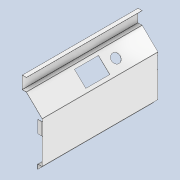
# Autodesk Inventor part: Carcaza_blanca_frontal
Saved by Autodesk Inventor 2021 (Build 250183000, 183)
## iProperties
Created: 2021-04-15
Part Number: Carcaza_blanca_frontal
Material: Genérico
Document SubType Name: Chapa
Designer: Admin
Density: 1 g/cm^3
Sheet Metal Rule: Por defecto_mm
Appearance: Blanco
Author: Admin
Autodesk Inventor part; units mm, degrees
ref_plane "YZ Plane" through (0, 0, 0) normal (1, 0, 0) x (0, 1, 0)
ref_plane "XZ Plane" through (0, 0, 0) normal (0, 1, 0) x (-1, 0, 0)
ref_plane "XY Plane" through (0, 0, 0) normal (0, 0, 1) x (1, 0, 0)
sketch "Boceto1" plane through (0, 0, 0) normal (1, 0, 0) x (0, 1, 0)
  line L0 (0, 0) -> (189.4, 0)
  line L1 (189.4, 0) -> (189.4, -527.58)
  line L2 (189.4, -527.58) -> (0, -527.58)
  line L3 (0, -527.58) -> (0, 0)
  dimension "d0" = 189.4
  dimension "d1" = 527.58
  measures "d0" distance of L1.end L2.end
  measures "d1" distance of L0.end L1.end
extrude "Placa1" add sketch "Boceto1" along normal blind 0.92
sketch "Boceto2" plane through (0.92, 0.92, -527.58) normal (0, -1, 0) x (-1, 0, 0)
  line L0 (0, 527.58) -> (0, 0)
  line L1 (0, 0) -> (21.6, 0)
  line L2 (21.6, 0) -> (21.6, 527.58)
  line L3 (21.6, 527.58) -> (0, 527.58)
  constraints: 6 end point, 1 horizontal, 1 perpendicular, 1 vertical
edge flange "Pestaña1" height 21.6 angle 90 thickness 0.92 bend radius 0.92 thickness toward (0, -1, 0) relief straight relief width 0.92 relief depth 0.46 edges at (0.92, 0, -263.79) wall of the first edge with corners at (0.92, 0.92, 0) (0.92, 0.92, -527.58) (-20.68, 0.92, -527.58) (-20.68, 0.92, 0)
bend "Doblez1"
corner "Esquina1"
sketch "Boceto3" plane through (-19.76, 0.92, 0) normal (-1, 0, 0) x (0, 1, 0)
  line L0 (0, -527.58) -> (0, 0)
  line L1 (0, 0) -> (-21.6, 0)
  line L2 (-21.6, 0) -> (-21.6, -527.58)
  line L3 (-21.6, -527.58) -> (0, -527.58)
  constraints: 8 end point
edge flange "Pestaña2" height 21.6 angle 90 thickness 0.92 bend radius 0.92 thickness toward (-1, 0, 0) relief straight relief width 0.92 relief depth 0.46 edges at (-20.68, 0.92, -263.79) wall of the first edge with corners at (-19.76, 0.92, -527.58) (-19.76, 0.92, 0) (-19.76, -20.68, 0) (-19.76, -20.68, -527.58)
bend "Doblez2"
corner "Esquina2"
sketch "Boceto4" plane through (0.2822, 188.737, 0) normal (0.6932761, 0.7206721, 0) x (0.7206721, -0.6932761, 0)
  line L0 (0, -527.58) -> (0, 0)
  line L1 (0, 0) -> (-100.563, 0)
  line L2 (-100.563, 0) -> (-100.563, -527.58)
  line L3 (-100.563, -527.58) -> (0, -527.58)
  constraints: 6 end point, 1 horizontal, 1 perpendicular, 1 vertical
edge flange "Pestaña3" height 100.563 angle 46.11 thickness 0.92 bend radius 0.92 thickness toward (0.6932761, 0.7206721, 0) relief straight relief width 0.92 relief depth 0.46 edges at (0.92, 189.4, -263.79) wall of the first edge with corners at (0.2822, 188.737, -527.58) (0.2822, 188.737, 0) (-72.1908, 258.4549, 0) (-72.1908, 258.4549, -527.58)
bend "Doblez3"
corner "Esquina3"
sketch "Boceto5" plane through (-71.553, 258.1979, 0) normal (0, 1, 0) x (1, 0, 0)
  line L0 (0, -527.58) -> (0, 0)
  line L1 (0, 0) -> (-20, 0)
  line L2 (-20, 0) -> (-20, -527.58)
  line L3 (-20, -527.58) -> (0, -527.58)
  constraints: 6 end point, 1 horizontal, 1 perpendicular, 1 vertical
edge flange "Pestaña4" height 20 angle 43.89 thickness 0.92 bend radius 0.92 thickness toward (0, 1, 0) relief straight relief width 0.92 relief depth 0.46 edges at (-71.553, 259.1179, -263.79) wall of the first edge with corners at (-71.553, 258.1979, -527.58) (-71.553, 258.1979, 0) (-91.553, 258.1979, 0) (-91.553, 258.1979, -527.58)
bend "Doblez4"
corner "Esquina4"
sketch "Boceto6" plane through (-90.633, 258.1979, 0) normal (-1, 0, 0) x (0, -1, 0)
  line L0 (0, -527.58) -> (0, 0)
  line L1 (0, 0) -> (-58.71, 0)
  line L2 (-58.71, 0) -> (-58.71, -527.58)
  line L3 (-58.71, -527.58) -> (0, -527.58)
  constraints: 6 end point, 1 horizontal, 1 perpendicular, 1 vertical
edge flange "Pestaña5" height 58.71 angle 90 thickness 0.92 bend radius 0.92 thickness toward (-1, 0, 0) relief straight relief width 0.92 relief depth 0.46 edges at (-91.553, 259.1179, -263.79) wall of the first edge with corners at (-90.633, 258.1979, -527.58) (-90.633, 258.1979, 0) (-90.633, 316.9079, 0) (-90.633, 316.9079, -527.58)
bend "Doblez5"
corner "Esquina5"
sketch "Boceto7" plane through (-91.553, 315.9879, -527.58) normal (0, 1, 0) x (1, 0, 0)
  line L0 (0, 527.58) -> (0, 0)
  line L1 (0, 0) -> (20, 0)
  line L2 (20, 0) -> (20, 527.58)
  line L3 (20, 527.58) -> (0, 527.58)
  constraints: 6 end point, 1 horizontal, 1 perpendicular, 1 vertical
edge flange "Pestaña6" height 20 angle 90 thickness 0.92 bend radius 0.92 thickness toward (0, 1, 0) relief straight relief width 0.92 relief depth 0.46 edges at (-91.553, 316.9079, -263.79) wall of the first edge with corners at (-91.553, 315.9879, 0) (-91.553, 315.9879, -527.58) (-71.553, 315.9879, -527.58) (-71.553, 315.9879, 0)
bend "Doblez6"
corner "Esquina6"
sketch "Boceto8" plane through (0, 1.84, 0) normal (0, 0, 1) x (1, 0, 0)
  line L0 (0.92, 186.7769) -> (0.92, 0)
  line L1 (0.92, 174.636) -> (-19.08, 174.636)
  line L2 (-19.08, 174.636) -> (-19.08, 118.6032)
  line L3 (-19.08, 118.6032) -> (0.92, 118.6032)
  line L4 (0.92, 118.6032) -> (0.92, 174.636)
  point P0 (0, -1.84)
  dimension "d63" = 20
  measures "d63" distance of L3.end L2.end
sheet face with bend "Cara2" sketch "Boceto8" thickness 0.92 toward (0, 0, -1) bend radius 0.92 relief straight relief width 0.92 relief depth 0.46
bend "Doblez7"
sketch "Boceto9" plane through (0, 1.84, -527.58) normal (0, 0, -1) x (-1, 0, 0)
  line L0 (-0.92, 174.636) -> (-0.92, 118.6032)
  line L1 (19.08, 174.636) -> (19.08, 118.6032)
  line L2 (-0.92, 174.636) -> (19.08, 174.636)
  line L3 (19.08, 174.636) -> (19.08, 118.6032)
  line L4 (19.08, 118.6032) -> (-0.92, 118.6032)
  line L5 (-0.92, 118.6032) -> (-0.92, 174.636)
  point P0 (0, -1.84)
sheet face with bend "Cara3" sketch "Boceto9" thickness 0.92 toward (0, 0, 1) bend radius 0.92 relief straight relief width 0.92 relief depth 0.46
bend "Doblez8"
sketch "Boceto10" plane through (0.3556, 189.9429, 0) normal (0.6932761, 0.7206721, 0) x (0.7206721, -0.6932761, 0)
  line L0 (0, 527.58) -> (0, 0) projected
  line L1 (-100.3142, 0) -> (-100.3142, 527.58) projected
  line L2 (-14, 263.79) -> (-14, 318.59)
  line L3 (-14, 318.59) -> (-85.6, 318.59)
  line L4 (-85.6, 318.59) -> (-85.6, 208.99)
  line L5 (-85.6, 208.99) -> (-14, 208.99)
  line L6 (-14, 208.99) -> (-14, 263.79)
  line L7 (-49.8, 263.79) -> (-49.8, 371.79)
  circle A0 centre (-49.8, 371.79) radius 20
  point P0 (131.4266, 0)
  dimension "d75" = 54.8
  dimension "d76" = 71.6
  dimension "d77" = 109.6
  dimension "d78" = 71.6
  dimension "d81" = 108
  dimension "d82" = 40
  constraints: 12 end point, 2 perpendicular, 1 centre point, 1 coincident, 1 point on line, 1 vertical
  measures "d75" distance of L2.start L2.end
  measures "d76" distance of L2.end L3.end
  measures "d77" distance of L3.end L4.end
  measures "d78" distance of L4.end L5.end
  measures "d81" distance of L7.start L7.end
  measures "d82" diameter of A0
extrude "Extrusión1" cut sketch "Boceto10" against normal blind 10
equation "\"d2\" = Grosor"
equation "\"d3\" = Anchura_desahogo_plegado"
equation "\"d4\" = Profundidad_desahogo_plegado"
equation "\"d5\" = Remanente_mínimo"
equation "\"d6\" = Radiodetransición"
equation "\"d9\" = Radio_pliegue"
equation "\"d10\" = Tamaño_destalonado"
equation "\"d11\" = TamañoSeparación"
equation "\"d12\" = Tamaño_de_radio_de_Jacobi"
equation "\"d13\" = Anchura_desahogo_plegado"
equation "\"d14\" = Profundidad_desahogo_plegado"
equation "\"d15\" = Remanente_mínimo"
equation "\"d16\" = Radiodetransición"
equation "\"d19\" = Radio_pliegue"
equation "\"d20\" = Tamaño_destalonado"
equation "\"d21\" = TamañoSeparación"
equation "\"d22\" = Tamaño_de_radio_de_Jacobi"
equation "\"d23\" = Anchura_desahogo_plegado"
equation "\"d24\" = Profundidad_desahogo_plegado"
equation "\"d25\" = Remanente_mínimo"
equation "\"d26\" = Radiodetransición"
equation "\"d29\" = Radio_pliegue"
equation "\"d30\" = Tamaño_destalonado"
equation "\"d31\" = TamañoSeparación"
equation "\"d32\" = Tamaño_de_radio_de_Jacobi"
equation "\"d33\" = Anchura_desahogo_plegado"
equation "\"d34\" = Profundidad_desahogo_plegado"
equation "\"d35\" = Remanente_mínimo"
equation "\"d36\" = Radiodetransición"
equation "\"d39\" = Radio_pliegue"
equation "\"d40\" = Tamaño_destalonado"
equation "\"d41\" = TamañoSeparación"
equation "\"d42\" = Tamaño_de_radio_de_Jacobi"
equation "\"d43\" = Anchura_desahogo_plegado"
equation "\"d44\" = Profundidad_desahogo_plegado"
equation "\"d45\" = Remanente_mínimo"
equation "\"d46\" = Radiodetransición"
equation "\"d49\" = Radio_pliegue"
equation "\"d50\" = Tamaño_destalonado"
equation "\"d51\" = TamañoSeparación"
equation "\"d52\" = Tamaño_de_radio_de_Jacobi"
equation "\"d53\" = Anchura_desahogo_plegado"
equation "\"d54\" = Profundidad_desahogo_plegado"
equation "\"d55\" = Remanente_mínimo"
equation "\"d56\" = Radiodetransición"
equation "\"d59\" = Radio_pliegue"
equation "\"d60\" = Tamaño_destalonado"
equation "\"d61\" = TamañoSeparación"
equation "\"d62\" = Tamaño_de_radio_de_Jacobi"
equation "\"d64\" = Radio_pliegue"
equation "\"d65\" = Anchura_desahogo_plegado"
equation "\"d67\" = Remanente_mínimo"
equation "\"d66\" = Profundidad_desahogo_plegado"
equation "\"d68\" = Radiodetransición"
equation "\"d69\" = Radio_pliegue"
equation "\"d70\" = Anchura_desahogo_plegado"
equation "\"d72\" = Remanente_mínimo"
equation "\"d71\" = Profundidad_desahogo_plegado"
equation "\"d73\" = Radiodetransición"
equation "\"Radio_pliegue\" = Grosor"
equation "\"Anchura_desahogo_plegado\" = Grosor"
equation "\"Profundidad_desahogo_plegado\" = 0.5 * Grosor"
equation "\"Tamaño_destalonado\" = 4 * Grosor"
equation "\"Remanente_mínimo\" = 2 * Grosor"
equation "\"Radiodetransición\" = Radio_pliegue"
equation "\"Tamaño_de_radio_de_Jacobi\" = Radio_pliegue"
equation "\"TamañoSeparación\" = Grosor"
equation "\"Grosor\" = 0.92"
